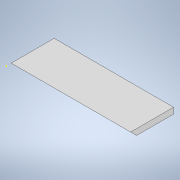
# Autodesk Inventor part: Helenowiak_plug
Saved by Autodesk Inventor 2021 (Build 250183000, 183)
## iProperties
Created: 2021-03-30
Part Number: Helenowiak_plug
Material: Ogólny
Document SubType Name: Modeling
Designer: jakub
Density: 1 g/cm^3
Appearance: Domyślna
Author: jakub
Autodesk Inventor part; units mm, degrees
ref_plane "YZ Plane" through (0, 0, 0) normal (1, 0, 0) x (0, 1, 0)
ref_plane "XZ Plane" through (0, 0, 0) normal (0, 1, 0) x (-1, 0, 0)
ref_plane "XY Plane" through (0, 0, 0) normal (0, 0, 1) x (1, 0, 0)
sketch "Szkic1" plane through (0, 0, 0) normal (0, 1, 0) x (-1, 0, 0)
  line L0 (0, 0) -> (-100, 0)
  line L1 (-100, 0) -> (-100, -40)
  line L2 (-100, -40) -> (0, -40)
  line L3 (0, -40) -> (0, 0)
  dimension "d0" = 100
  dimension "d1" = 40
  constraints: 8 end point, 2 parallel, 1 horizontal, 1 perpendicular
  measures "d0" distance of L2.end L1.end
  measures "d1" distance of L1.end L0.end
extrude "Wyciągnięcie proste1" add sketch "Szkic1" along normal blind 5
sketch "Szkic4" plane through (100, 0, 0) normal (1, 0, 0) x (0, 0, -1)
  line L0 (0, 5) -> (40, 5) projected
  line L1 (0, 5) -> (4.346, 0)
  line L2 (0, 0) -> (40, 0) projected
  line L3 (0, 0) -> (0, 5) projected
  line L4 (0, 0) -> (0, 5)
  line L5 (0, 5) -> (4.346, 0)
  constraints: 6 end point, 2 collinear, 1 point on line
extrude "Wyciągnięcie proste2" cut sketch "Szkic4" against normal blind 100
sketch "Szkic5" plane through (100, 0, -40) normal (1, 0, 0) x (0, 0, -1)
  line L0 (-40, 5) -> (0, 5) projected
  line L1 (-40, 5) -> (-35, 0)
  line L2 (-35.654, 0) -> (0, 0) projected
  line L3 (-40, 5) -> (-32.9289, 5) construction
  line L4 (-35, 0) -> (-40, 0)
  line L5 (-35.654, 0) -> (-40, 5) projected
  line L6 (-40, 0) -> (-40, 5)
  dimension "d6" = 45
  constraints: 8 end point, 1 collinear, 1 equal length, 1 horizontal, 1 perpendicular, 1 point on line
  measures "d6" angle of L1 L3
extrude "Wyciągnięcie proste3" cut sketch "Szkic5" against normal blind 100.25
sketch "Szkic6" plane through (100, 0, -40) normal (1, 0, 0) x (0, 0, -1)
  line L0 (0, 5) -> (-40, 5) projected
  line L1 (-40, 5) -> (-38, 5)
  line L2 (-38, 5) -> (-33, 0)
  line L3 (0, 0) -> (-35, 0) projected
  line L4 (-33, 0) -> (-35, 0)
  line L5 (-35, 0) -> (-40, 5)
  point P0 (-40, 0)
  dimension "d9" = 2
  dimension "d10" = 135
  constraints: 8 end point, 2 point on line, 1 collinear
  measures "d9" distance of L0.end L1.end
  measures "d10" angle of L1 L2
extrude "Wyciągnięcie proste4" cut sketch "Szkic6" against normal blind 100.25
sketch "Szkic7" plane through (100, 0, -40) normal (1, 0, 0) x (0, 0, -1)
  line L0 (-33, 0) -> (-38, 5) projected
  line L1 (-38, 5) -> (-36, 5)
  line L2 (0, 5) -> (-38, 5) projected
  line L3 (-36, 5) -> (-31, 0)
  line L4 (0, 0) -> (-33, 0) projected
  line L5 (-31, 0) -> (-33, 0)
  line L6 (-33, 0) -> (-38, 5)
  point P0 (-40, 0)
  dimension "d13" = 2
  dimension "d14" = 135
  constraints: 8 end point, 2 point on line, 1 collinear, 1 parallel
  measures "d13" distance of L0.end L1.end
  measures "d14" angle of L1 L3
extrude "Wyciągnięcie proste5" cut sketch "Szkic7" against normal blind 100
sketch "Szkic11" plane through (0, 5, 0) normal (0, 1, 0) x (1, 0, 0)
  point P0 (0, 0)
